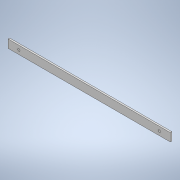
# Autodesk Inventor part: 零件1
Saved by Autodesk Inventor 2022 (Build 260153000, 153)
## iProperties
Created: 2023-04-16
Part Number: 零件1
Material: 一般
Document SubType Name: Modeling
Designer: JOU
Density: 1 g/cm^3
Appearance: 預設
Author: JOU
Autodesk Inventor part; units mm, degrees
ref_plane "YZ Plane" through (0, 0, 0) normal (1, 0, 0) x (0, 1, 0)
ref_plane "XZ Plane" through (0, 0, 0) normal (0, 1, 0) x (-1, 0, 0)
ref_plane "XY Plane" through (0, 0, 0) normal (0, 0, 1) x (1, 0, 0)
sketch "草圖1" plane through (0, 0, 0) normal (0, 0, 1) x (1, 0, 0)
  line L0 (0, 15) -> (300, 15)
  line L1 (300, 15) -> (300, 0)
  line L2 (300, 0) -> (0, 0)
  line L3 (0, 0) -> (0, 15)
  circle A0 centre (20, 7.5) radius 2
  circle A1 centre (280, 7.5) radius 2
  dimension "d0" = 300
  dimension "d1" = 15
  dimension "d2" = 7.5
  dimension "d3" = 4
  dimension "d4" = 20
  dimension "d5" = 20
  dimension "d6" = 7.5
  dimension "d7" = 4
  constraints: 8 end point, 2 centre point, 2 parallel, 1 coincident, 1 horizontal, 1 perpendicular
  measures "d0" distance of L0.start L0.end
  measures "d1" distance of L2.end L0.start
  measures "d2" distance from line of L0 A0.centre
  measures "d3" diameter of A0
  measures "d4" distance from line of L3 A0.centre
  measures "d5" distance from line of A1.centre L1
  measures "d6" distance from line of L0 A1.centre
  measures "d7" diameter of A1
extrude "擠出1" add sketch "草圖1" along normal blind 3
